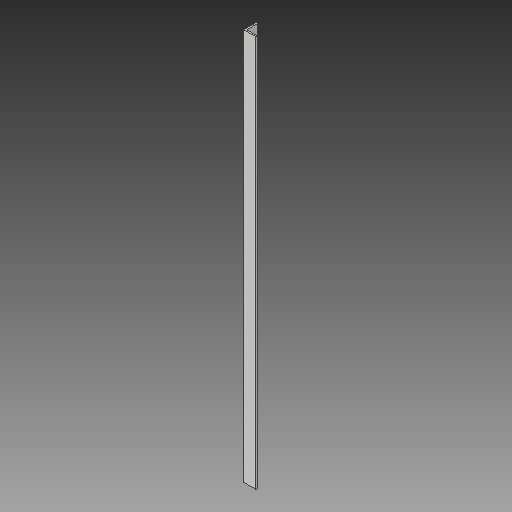
# Autodesk Inventor part: BumperMount1-ver1-1111-2019
Saved by Autodesk Inventor 2018 (Build 220112000, 112)
## iProperties
Created: 2020-01-11
Part Number: BumperMount1-ver1-1111-2019
Material: Generic
Document SubType Name: Modeling
Designer: JMHal
Density: 1 g/cm^3
Appearance: Default
Author: JMHal
Autodesk Inventor part; units mm, degrees
ref_plane "YZ Plane" through (0, 0, 0) normal (1, 0, 0) x (0, 1, 0)
ref_plane "XZ Plane" through (0, 0, 0) normal (0, 1, 0) x (-1, 0, 0)
ref_plane "XY Plane" through (0, 0, 0) normal (0, 0, 1) x (1, 0, 0)
sketch "Sketch3" plane through (0, 0, 0) normal (0, 1, 0) x (-1, 0, 0)
  line L0 (0, 0) -> (25.4, 0)
  line L1 (25.4, 0) -> (25.4, -3.175)
  line L2 (25.4, -3.175) -> (0, -3.175)
  line L3 (0, -3.175) -> (0, 0)
  line L4 (25.4, 0) -> (22.225, 0)
  line L5 (22.225, 0) -> (22.225, -25.4)
  line L6 (22.225, -25.4) -> (25.4, -25.4)
  line L7 (25.4, -25.4) -> (25.4, 0)
  dimension "d8" = 25.4
  dimension "d9" = 3.175
  dimension "d10" = 3.175
  dimension "d11" = 25.4
  constraints: 16 end point, 4 parallel, 2 horizontal, 2 perpendicular
  measures "d8" distance of L1.end L2.end
  measures "d9" distance between parallel lines of L2 L0
  measures "d10" distance between parallel lines of L5 L7
  measures "d11" distance between parallel lines of L6 L0
extrude "Extrusion3" add sketch "Sketch3" along normal blind 812.8
body "Solid3"
